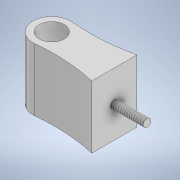
# Autodesk Inventor part: backupstability
Saved by Autodesk Inventor 2020 (Build 240168000, 168)
## iProperties
Created: 2019-07-11
Part Number: backupstability
Material: Generic
Document SubType Name: Modeling
Designer: ColinP
Density: 1 g/cm^3
Appearance: Default
Author: ColinP
Autodesk Inventor part; units mm, degrees
ref_plane "YZ Plane" through (0, 0, 0) normal (1, 0, 0) x (0, 1, 0)
ref_plane "XZ Plane" through (0, 0, 0) normal (0, 1, 0) x (-1, 0, 0)
ref_plane "XY Plane" through (0, 0, 0) normal (0, 0, 1) x (1, 0, 0)
sketch "Sketch1" plane through (0, 0, 0) normal (0, 1, 0) x (-1, 0, 0)
  line L0 (0, 0) -> (28.575, 0)
  line L1 (28.575, 0) -> (0, 0)
  line L2 (0, 0) -> (-14.2875, -24.7467)
  line L3 (0, 0) -> (28.575, 0) construction
  line L4 (0, 0) -> (-14.2875, 24.7467)
  line L5 (0, 0) -> (28.575, 0) construction
  circle A0 centre (28.575, 0) radius 2.54
  circle A1 centre (-14.2875, -24.7467) radius 2.54
  circle A2 centre (-14.2875, 24.7467) radius 2.54
  circle A3 centre (0, 0) radius 3.175
  circle A4 centre (0, 0) radius 6.35
  line L6 (-1.5875, -2.7496) -> (0, 0)
  line L7 (0, 0) -> (-6.35, 0)
  circle A5 centre (-14.2875, 24.7467) radius 3.81
  circle A6 centre (28.575, 0) radius 3.81
  circle A7 centre (-14.2875, -24.7467) radius 3.81
  line L8 (30.6811, 3.175) -> (-12.1814, 27.9217)
  line L9 (28.2054, -3.792) -> (-10.8187, -26.3226)
  line L10 (-18.0975, 24.7467) -> (-18.0975, -24.7467)
  line L11 (0, 0) -> (5.0525, -8.8146)
  line L12 (0, 0) -> (5.1463, 8.7602)
  line L13 (0, 0) -> (-10.16, 0)
  arc A8 (28.2054, -3.792) -> (-10.8187, -26.3226) centre (24.4473, -42.344) ccw
  arc A9 (-10.8187, 26.3226) -> (28.2054, 3.792) centre (24.4473, 42.344) ccw
  arc A10 (-17.3867, -22.5305) -> (-17.3867, 22.5305) centre (-48.8947, 0) ccw
  point P0 (5.1074, 8.7829)
  point P1 (-10.16, 0.0317)
  point P2 (30.2716, 3.4114)
  point P3 (28.2054, 3.792)
  point P4 (-10.8187, 26.3226)
  point P5 (-17.3867, 22.5305)
  point P6 (-17.3867, -22.5305)
  dimension "d9" = 6.35
  dimension "d41" = 12.7
  dimension "d0" = 28.575
  dimension "d1" = 28.575
  dimension "d2" = 120
  dimension "d3" = 28.575
  dimension "d4" = 120
  dimension "d5" = 5.08
  dimension "d6" = 5.08
  dimension "d7" = 5.08
  dimension "d42" = 7.62
  dimension "d43" = 7.62
  dimension "d44" = 7.62
  dimension "d47" = 10.16
  dimension "d48" = 10.16
  dimension "d49" = 10.16
  dimension "d52" = 360
  constraints: 28 end point, 15 point on circle, 9 centre point, 8 coincident, 4 horizontal, 3 tangent, 2 collinear, 2 equal length, 2 point on line, 1 horizontal alignment, 21 other
  measures "d0" distance of L0.start L0.end
  measures "d1" distance of L0.start L2.end
  measures "d2" angle of L2 L3
  measures "d3" distance of L0.start L4.end
  measures "d4" angle of L5 L4
  measures "d5" diameter of A0
  measures "d6" diameter of A1
  measures "d7" diameter of A2
  measures "d42" diameter of A5
  measures "d43" diameter of A6
  measures "d44" diameter of A7
  measures "d47" distance of L6.end L11.end
  measures "d48" distance of L6.end L12.end
  measures "d49" distance of L6.end L13.end
extrude "Extrusion4" add sketch "Sketch1" along normal blind 12.7 contours A3 L12 A4 L0 | L0 A4 L11 A3 | A3 L11 A4 L2 | L2 A4 L7 A3 | A3 L7 A4 L4 | L4 A4 L12 A3 | A4 L12 A9 A6 L0 | L0 A6 A8 L11 A4 | A4 L11 A8 A7 L2 | L2 A7 A10 L13 A4 | A4 L13 A10 A5 L4 | L4 A5 A9 L12 A4 | A6 L8 | A7 | A5 picked at (31.8987, 0.5122)
sketch "Sketch8" plane through (0, 12.7, 0) normal (0, 1, 0) x (1, 0, 0)
  circle A0 centre (0.678, -11.6167) radius 3.175 projected
  circle A1 centre (9.1268, -7.2186) radius 3.175 projected
  circle A2 centre (0.678, -11.6167) radius 3.175 projected
  circle A3 centre (9.1268, -7.2186) radius 3.175 projected
  line L0 (5.0649, -17.2561) -> (12.4117, -13.0144)
  arc A4 (17.3867, 22.5305) -> (17.3867, -22.5305) centre (48.8947, 0) ccw projected
  circle A5 centre (14.2875, -24.7467) radius 2.54 projected
  line L1 (0, 0) -> (14.2875, -24.7467)
  arc A6 (10.8187, -26.3226) -> (-28.2054, -3.792) centre (-24.4473, -42.344) ccw projected
  arc A7 (10.8187, -26.3226) -> (17.3867, -22.5305) centre (14.2875, -24.7467) ccw projected
  line L2 (9.1268, -7.2186) -> (10.7143, -9.9682)
  line L3 (9.1268, -7.2186) -> (7.5393, -4.4689)
  line L4 (0.678, -11.6167) -> (-0.9095, -8.867)
  line L5 (0.678, -11.6167) -> (2.2655, -14.3663)
  line L6 (-0.9095, -8.867) -> (-4.4671, -10.921)
  line L7 (2.2655, -14.3663) -> (-2.6369, -17.1967)
  line L8 (7.5393, -4.4689) -> (12.4407, -1.6391)
  line L9 (10.7143, -9.9682) -> (17.8581, -5.8438)
  point P0 (11.3663, -9.5918)
  point P1 (11.3414, -9.4937)
  point P2 (10.4005, -4.3102)
  point P3 (10.2682, -2.8934)
  point P4 (-0.9095, -8.867)
  point P5 (-3.012, -10.0809)
  point P6 (2.1732, -14.2063)
  constraints: 20 end point, 6 point on circle, 5 perpendicular, 2 parallel, 2 point on line, 2 tangent
extrude "Extrusion5" cut sketch "Sketch8" against normal through all contours A0 A6 L5 L4 | L4 L5 A6 A0 | A0 A6 L6 | A0 L5 A6 | L3 L2 A1 | L8 A4 A1 | A1 A4 L2 L3 | A1 A4 L9 | A1 A4 picked at (2.2194, -14.2744)
sketch "Sketch11" plane through (0, 12.7, 0) normal (0, 1, 0) x (1, 0, 0)
  arc A0 (10.8187, -26.3226) -> (2.3124, -14.3387) centre (-24.4473, -42.344) ccw projected
  arc A1 (11.3663, -9.5918) -> (17.3867, -22.5305) centre (48.8947, 0) ccw projected
  arc A2 (10.8187, -26.3226) -> (17.3867, -22.5305) centre (14.2875, -24.7467) ccw projected
  line L0 (0, 0) -> (14.2875, -24.7467)
  circle A3 centre (14.2875, -24.7467) radius 2.54 projected
  line L1 (14.2875, -24.7467) -> (8.2579, -14.3032)
  line L2 (14.2875, -24.7467) -> (7.9375, -13.7482)
  line L3 (7.9375, -13.7482) -> (11.895, -11.4633)
  line L4 (7.9375, -13.7482) -> (3.98, -16.033)
  circle A4 centre (14.2875, 24.7467) radius 2.54 projected
  line L5 (0, 0) -> (14.2875, 24.7467)
  line L6 (14.2875, 24.7467) -> (7.9375, 13.7482)
  line L7 (7.9375, 13.7482) -> (0, 0)
  circle A5 centre (-28.575, 0) radius 2.54 projected
  line L8 (0, 0) -> (-28.575, 0)
  line L9 (-28.575, 0) -> (-15.875, 0)
  line L10 (-15.875, 0) -> (-15.875, 4.5698)
  arc A6 (-28.2054, 3.792) -> (10.8187, 26.3226) centre (-24.4473, 42.344) ccw projected
  line L11 (-15.875, 0) -> (-15.875, -4.5698)
  line L12 (7.9375, 13.7482) -> (3.98, 16.033)
  line L13 (7.9375, 13.7482) -> (11.895, 11.4633)
  arc A7 (17.3867, 22.5305) -> (10.2682, -2.8934) centre (48.8947, 0) ccw projected
  arc A8 (-28.2054, 3.792) -> (-30.6811, -3.175) centre (-28.575, 0) ccw projected
  arc A9 (-3.012, -10.0809) -> (-28.2054, -3.792) centre (-24.4473, -42.344) ccw projected
  arc A10 (-30.2716, -3.4114) -> (-28.2054, -3.792) centre (-28.575, 0) ccw projected
  line L14 (-30.6811, -3.175) -> (-30.2716, -3.4114) projected
  arc A11 (17.3867, 22.5305) -> (10.8187, 26.3226) centre (14.2875, 24.7467) ccw projected
  line L15 (-3.012, -10.0809) -> (-0.9095, -8.867) projected
  arc A12 (2.3124, -14.3387) -> (-0.9095, -8.867) centre (0.678, -11.6167) ccw projected
  arc A13 (7.5393, -4.4689) -> (10.7143, -9.9682) centre (9.1268, -7.2186) ccw projected
  line L16 (11.3663, -9.5918) -> (10.7143, -9.9682) projected
  line L17 (7.5393, -4.4689) -> (10.2682, -2.8934) projected
  dimension "d65" = 12.7
  dimension "d66" = 12.7
  dimension "d67" = 12.7
  constraints: 28 end point, 7 point on line, 5 point on circle, 3 perpendicular, 1 horizontal
  measures "d65" distance of L1.start L2.end
  measures "d66" distance of L5.end L6.end
  measures "d67" distance of L8.end L9.end
extrude "Extrusion6" cut sketch "Sketch11" against normal blind 12.7 contours A0 A12 L15 A9 L11 L8 L0 L4 | L0 L5 L13 A7 L17 A13 L16 A1 L3 | L8 L10 A6 L12 L5
sketch "Sketch13" plane through (0, 12.7, 0) normal (0, 1, 0) x (1, 0, 0)
  arc A0 (-28.2054, 3.792) -> (-15.875, 4.5698) centre (-24.4473, 42.344) ccw projected
  arc A1 (-15.875, -4.5698) -> (-28.2054, -3.792) centre (-24.4473, -42.344) ccw projected
  line L0 (-15.875, -4.5698) -> (-15.875, 4.5698) projected
  arc A2 (-30.2716, -3.4114) -> (-28.2054, -3.792) centre (-28.575, 0) ccw projected
  arc A3 (-28.2054, 3.792) -> (-30.6811, -3.175) centre (-28.575, 0) ccw projected
  arc A4 (17.3867, 22.5305) -> (11.895, 11.4633) centre (48.8947, 0) ccw projected
  line L1 (3.98, 16.033) -> (11.895, 11.4633) projected
  arc A5 (3.98, 16.033) -> (10.8187, 26.3226) centre (-24.4473, 42.344) ccw projected
  arc A6 (17.3867, 22.5305) -> (10.8187, 26.3226) centre (14.2875, 24.7467) ccw projected
  arc A7 (11.895, -11.4633) -> (17.3867, -22.5305) centre (48.8947, 0) ccw projected
  line L2 (11.895, -11.4633) -> (3.98, -16.033) projected
  arc A8 (10.8187, -26.3226) -> (3.98, -16.033) centre (-24.4473, -42.344) ccw projected
  arc A9 (10.8187, -26.3226) -> (17.3867, -22.5305) centre (14.2875, -24.7467) ccw projected
  point P0 (0, 0)
extrude "Extrusion7" cut sketch "Sketch13" against normal blind 12.7
sketch "Sketch14" plane through (-15.875, 12.7, 4.5698) normal (1, 0, 0) x (0, 0, -1)
  line L0 (0, -12.7) -> (0, 0) projected
  line L1 (0, -6.35) -> (9.1395, -6.35)
  line L2 (9.1395, 0) -> (9.1395, -12.7) projected
  line L3 (2.0298, 0) -> (7.1098, 0) projected
  line L4 (4.5698, 0) -> (4.5698, -12.7)
  circle A0 centre (4.5698, -6.35) radius 0.7876
  constraints: 4 end point, 4 midpoint, 1 centre point, 1 coincident, 1 vertical
extrude "Extrusion8" add sketch "Sketch14" along normal blind 6.6294
thread "Thread1" size "2-56 UNC" class "2A" standard "ANSI Unified Screw Threads" full length
ref_plane "Work Plane1" through (-32.385, 0, 0) normal (1, 0, 0) x (0, 1, 0)
sketch "Sketch23" plane through (-32.385, 0, 0) normal (1, 0, 0) x (0, 1, 0)
  point P0 (0, 0)
  point P1 (5.1729, 0.2292)
hole "Hole5" at (-32.385, 5.1729, 0.2292) direction (1, 0, 0) diameter 1.4211 depth 5.715 thread size "M1.8x0.35" class "6H" standard "ISO Metric profile"
body "Solid3"
